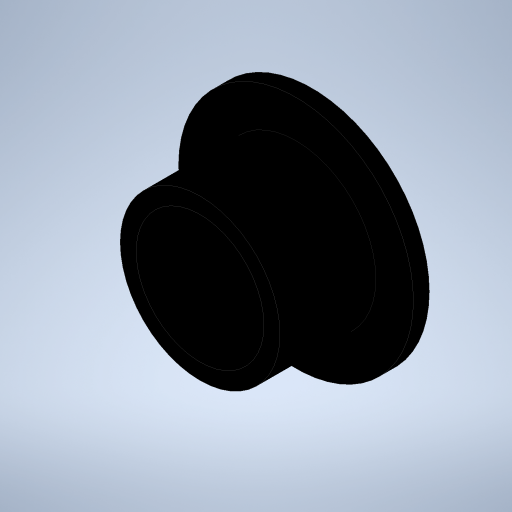
# Autodesk Inventor part: oilressbush8_10_sa
Saved by Autodesk Inventor 2024.1 (Build 281209000, 209)
## iProperties
Created: 2018-03-04
Part Number: oilressbush8_10_sa
Material: PC/ABS プラスチック
Document SubType Name: Modeling
Designer: shun
Density: 0.357273 g/cm^3
Appearance: 陽極酸化 - 黒
Author: shun
Autodesk Inventor part; units mm, degrees
ref_plane "YZ Plane" through (0, 0, 0) normal (1, 0, 0) x (0, 1, 0)
ref_plane "XZ Plane" through (0, 0, 0) normal (0, 1, 0) x (-1, 0, 0)
ref_plane "XY Plane" through (0, 0, 0) normal (0, 0, 1) x (1, 0, 0)
sketch "スケッチ1" plane through (0, 0, 0) normal (0, 0, 1) x (1, 0, 0)
  line L0 (4, 0) -> (7.35, 0)
  line L1 (7.35, 0) -> (7.35, -1)
  line L2 (7.35, -1) -> (5, -1)
  line L3 (5, -1) -> (5, -7)
  line L4 (5, -7) -> (4, -7)
  line L5 (4, -7) -> (4, 0)
  line L6 (0, -8.4) -> (0, 1.4) projected
  point P0 (0, 0)
  dimension "d0" = 4
  dimension "d2" = 1
  dimension "d3" = 2.35
  dimension "d4" = 6
  dimension "d5" = 90
  dimension "d6" = 1
  constraints: 12 end point, 4 perpendicular, 2 horizontal
  measures "d0" distance of point (0, 0) L0.start
  measures "d2" distance of L0.end L1.end
  measures "d3" distance of L1.end L2.end
  measures "d4" distance of L2.end L3.end
  measures "d5" angle of L3 L2
  measures "d6" distance of L3.end L4.end
revolve "回転1" add sketch "スケッチ1" angle 360 about axis through (0, -10, 0) along (0, 1, 0)
